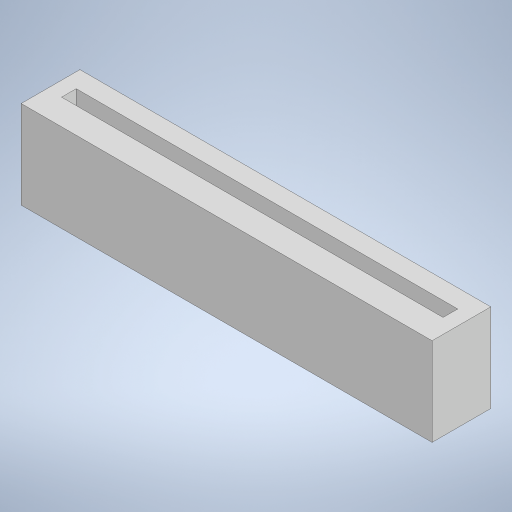
# Autodesk Inventor part: Better Breakout
Saved by Autodesk Inventor 2024.1 (Build 281209000, 209)
## iProperties
Created: 2024-01-16
Part Number: Better Breakout
Material: Generic
Document SubType Name: Modeling
Designer: ryanm
Density: 1 g/cm^3
Appearance: Default
Author: ryanm
Autodesk Inventor part; units mm, degrees
ref_plane "YZ Plane" through (0, 0, 0) normal (1, 0, 0) x (0, 1, 0)
ref_plane "XZ Plane" through (0, 0, 0) normal (0, 1, 0) x (-1, 0, 0)
ref_plane "XY Plane" through (0, 0, 0) normal (0, 0, 1) x (1, 0, 0)
sketch "Sketch1" plane through (0, 0, 0) normal (0, 1, 0) x (-1, 0, 0)
  line L0 (28, -4) -> (-28, -4)
  line L1 (-28, -4) -> (-28, 4)
  line L2 (-28, 4) -> (28, 4)
  line L3 (28, 4) -> (28, -4)
  point P0 (0, 0)
  point P1 (0, -4)
  point P2 (28, 0)
  dimension "d1" = 56
  dimension "d2" = 8
  constraints: 8 end point, 2 midpoint, 2 parallel, 1 horizontal, 1 horizontal alignment, 1 perpendicular, 1 vertical alignment
  measures "d1" distance of L0.start L0.end
  measures "d2" distance of L2.end L0.start
extrude "Extrusion1" add sketch "Sketch1" along normal blind 12
sketch "Sketch2" plane through (0, 12, 0) normal (0, 1, 0) x (1, 0, 0)
  line L0 (-26, 1.5) -> (26, 1.5)
  line L1 (26, 1.5) -> (26, -0.5)
  line L2 (26, -0.5) -> (-26, -0.5)
  line L3 (-26, -0.5) -> (-26, 1.5)
  line L4 (28, 4) -> (-28, 4) projected
  line L5 (28, -4) -> (28, 4) projected
  point P0 (0, 0)
  point P1 (0, 1.5)
  dimension "d5" = 2.5
  dimension "d6" = 2
  dimension "d7" = 2
  constraints: 8 end point, 2 parallel, 1 horizontal, 1 midpoint, 1 perpendicular, 1 vertical alignment
  measures "d5" distance between parallel lines of L0 L4
  measures "d6" distance of L2.end L0.start
  measures "d7" distance between parallel lines of L5 L1
extrude "Extrusion2" cut sketch "Sketch2" against normal blind 8.6
sketch "Sketch3" plane through (0, 3.4, 0) normal (0, 1, 0) x (1, 0, 0)
  line L0 (26, -0.5) -> (-26, -0.5) projected
  line L1 (26, 1.5) -> (26, -0.5) projected
  line L2 (-26, 1.5) -> (26, 1.5) projected
  line L3 (-26, -0.5) -> (-26, 1.5) projected
  line L4 (-25, 1.5) -> (-25, -0.5)
  line L5 (25, 1.5) -> (25, -0.5)
  point P0 (0, 0)
  dimension "d10" = 1
  dimension "d11" = 1
  constraints: 4 end point, 4 point on line, 1 perpendicular, 1 vertical
  measures "d10" distance between parallel lines of L4 L3
  measures "d11" distance between parallel lines of L1 L5
extrude "Extrusion3" cut sketch "Sketch3" against normal through all contours L0 L4 L2 L5
equation "\"d11\" = d10"
body "Solid1"
